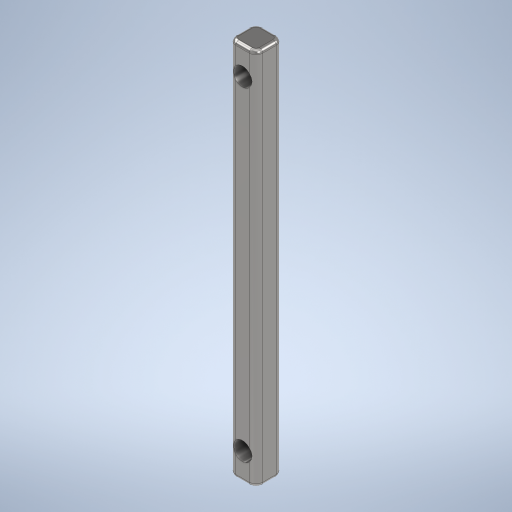
# Autodesk Inventor part: 45 stop
Saved by Autodesk Inventor 2023 (Build 270158000, 158)
## iProperties
Created: 2022-09-27
Part Number: 45 stop
Material: Stainless Steel
Document SubType Name: Modeling
Designer: aaron
Density: 8 g/cm^3
Appearance: Semi-Polished
Author: aaron
Autodesk Inventor part; units mm, degrees
ref_plane "YZ Plane" through (0, 0, 0) normal (1, 0, 0) x (0, 1, 0)
ref_plane "XZ Plane" through (0, 0, 0) normal (0, 1, 0) x (-1, 0, 0)
ref_plane "XY Plane" through (0, 0, 0) normal (0, 0, 1) x (1, 0, 0)
sketch "Sketch1" plane through (0, 0, 0) normal (0, 1, 0) x (-1, 0, 0)
  line L0 (-3.175, -3.175) -> (3.175, -3.175)
  line L1 (3.175, -3.175) -> (3.175, 3.175)
  line L2 (3.175, 3.175) -> (-3.175, 3.175)
  line L3 (-3.175, 3.175) -> (-3.175, -3.175)
  line L4 (-3.175, -3.175) -> (3.175, 3.175) construction
  line L5 (3.175, -3.175) -> (-3.175, 3.175) construction
  point P0 (0, 0)
  dimension "d0" = 6.35
  dimension "d1" = 6.35
  constraints: 12 end point, 2 midpoint, 2 parallel, 1 horizontal, 1 perpendicular
  measures "d0" distance of L2.end L1.end
  measures "d1" distance of L1.end L0.end
extrude "Extrusion1" add sketch "Sketch1" along normal blind 88.9
sketch "Sketch2" plane through (-3.175, 0, 3.175) normal (0, 0, 1) x (1, 0, 0)
  circle A0 centre (3.175, 6.35) radius 2.159
  line L0 (0, 0) -> (6.35, 0) projected
  circle A1 centre (3.175, 82.55) radius 2.159
  line L1 (0, 88.9) -> (6.35, 88.9) projected
  point P0 (3.175, 0)
  dimension "d4" = 4.318
  dimension "d5" = 6.35
  dimension "d6" = 4.318
  dimension "d7" = 6.35
  constraints: 2 centre point
  measures "d4" diameter of A0
  measures "d5" distance from line of L0 A0.centre
  measures "d6" diameter of A1
  measures "d7" distance from line of L1 A1.centre
extrude "Extrusion2" cut sketch "Sketch2" against normal blind 88.9
fillet "Fillet1" radius 1.5875 4 edges at (3.175, 44.45, -3.175) (-3.175, 44.45, -3.175) (3.175, 44.45, 3.175) (-3.175, 44.45, 3.175)
fillet "Fillet2" radius 0.7937 16 edges at (2.71, 88.9, -2.71) (0, 88.9, -3.175) (-2.71, 88.9, -2.71) (-3.175, 88.9, 0) (-2.71, 88.9, 2.71) (0, 88.9, 3.175) (2.71, 88.9, 2.71) (3.175, 88.9, 0) (0, 0, -3.175) (-2.71, 0, -2.71) (-3.175, 0, 0) (-2.71, 0, 2.71) (0, 0, 3.175) (2.71, 0, 2.71) (3.175, 0, 0) (2.71, 0, -2.71)
body "Solid1"
